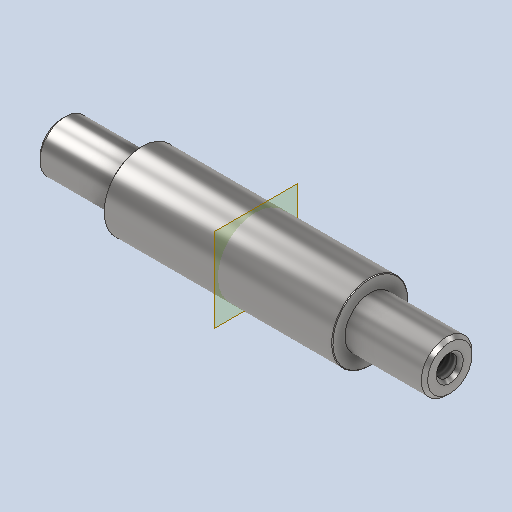
# Autodesk Inventor part: ParallelSystem_ProximalPart_Querstreben_v2_Rillenkugellager
Saved by Autodesk Inventor 2024 (Build 280153000, 153)
## iProperties
Created: 2022-07-19
Part Number: ParallelSystem_ProximalPart_Querstreben_v2_Rillenkugellager
Material: Edelstahl
Document SubType Name: Modeling
Designer: alexw
Density: 8 g/cm^3
Appearance: Halbpoliert
Mass: 41.3199 g
Surface Area: 23.7263 cm^2
Volume: 5.16499 cm^3
Author: alexw
Autodesk Inventor part; units mm, degrees
ref_plane "YZ Plane" through (0, 0, 0) normal (1, 0, 0) x (0, 1, 0)
ref_plane "XZ Plane" through (0, 0, 0) normal (0, 1, 0) x (-1, 0, 0)
ref_plane "XY Plane" through (0, 0, 0) normal (0, 0, 1) x (1, 0, 0)
sketch "Skizze1" plane through (0, 0, 0) normal (0, 0, 1) x (1, 0, 0)
  line L0 (0, 0) -> (0, 4)
  line L1 (0, 4) -> (12.5, 4)
  line L2 (12.5, 4) -> (12.5, 6)
  line L3 (12.5, 6) -> (48.5, 6)
  line L4 (48.5, 6) -> (48.5, 4)
  line L5 (48.5, 4) -> (61, 4)
  line L6 (61, 4) -> (61, 0)
  line L7 (61, 0) -> (0, 0)
  dimension "d1" = 12.5
  dimension "d2" = 12.5
  dimension "d3" = 8
  dimension "d4" = 12
  dimension "d29" = 36
  constraints: 16 end point, 6 perpendicular, 2 point on line, 1 vertical
  measures "d1" distance between parallel lines of L2 L0
  measures "d2" distance between parallel lines of L6 L4
  measures "d3" diameter of L1 L7
  measures "d4" diameter of L3 L7
  measures "d29" distance between parallel lines of L4 L2
revolve "Umdrehung1" add sketch "Skizze1" angle 360 about axis through (61, 0, 0) along (-1, 0, 0)
sketch "Skizze2" plane through (0, 0, 0) normal (-1, 0, 0) x (0, 0, 1)
  point P0 (0, 0)
  point P1 (0, 0)
  constraints: 1 coincident
sketch "Skizze3" plane through (61, 0, 0) normal (1, 0, 0) x (0, 0, -1)
  point P0 (0, 0)
  point P1 (0, 0)
  constraints: 1 coincident
hole "Bohrung1" at (61, 0, 0) direction (-1, 0, 0) diameter 3.242 depth 9 tip angle 118 thread size "M4x0.7" class "6H" standard "ISO Metric profile"
hole "Bohrung2" at (0, 0, 0) direction (1, 0, 0) diameter 3.242 depth 9 tip angle 118 thread size "M4x0.7" class "6H" standard "ISO Metric profile"
chamfer "Fase1" distance 0.5 angle 45 4 edges at (0, -4, 0) (61, -4, 0) (61, 0, 1.621) (0, 0, -1.621)
chamfer "Fase2" distance 0.1 angle 45 2 edges at (48.5, -6, 0) (12.5, -6, 0)
ref_plane "Arbeitsebene1" through (30.5, 0, 0) normal (-1, 0, 0) x (0, 0, 1)
equation "\"d1\" = d2"
equation "\"d29\" = MainAxis_Schluesselweite + 2 * ParallelMecha_Bearing_Step_Thickness"
equation "\"ParallelLink_BearingStep_Height\" = 5"
equation "\"ParallelMech_Distance_Step2Flat\" = 14"
equation "\"ParallelLink_Lever_Thickness_1\" = 8"
equation "\"ParallelMecha_Bearing_Step_Thickness\" = 6"
equation "\"MainAxis_Schluesselweite\" = 24"
